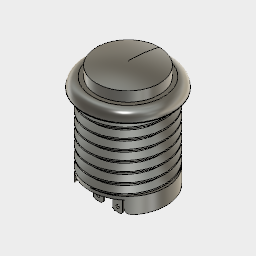
3429 Mini Arcade Button (Autodesk Fusion 360 design; units mm, degrees)
Autodesk Fusion 360 part; units mm, degrees
sketch "main circles" plane through (0, 0, 0) normal (0, 0, 1) x (1, 0, 0)
  circle A0 centre (0, 0) radius 12
  circle A1 centre (0, 0) radius 9.8
  circle A2 centre (0, 0) radius 13.8
  dimension "d1" = 24
  dimension "d2" = 19.6
  dimension "d3" = 27.6
  measures "d1" diameter of A0
  measures "d2" diameter of A1
  measures "d3" diameter of A2
extrude "Extrude1" add sketch "main circles" along normal blind 4.2 contours A1 makes body 1
sketch "curve revolve spline" plane through (0, 0, 0) normal (0, 1, 0) x (1, 0, 0)
  spline S0 degree 5 poles (0, -4.2) (-0.5903, -4.2) (-1.7268, -4.1833) (-3.2991, -4.1084) (-5.1578, -3.9245) (-7.1512, -3.617) (-8.4865, -3.3557) (-9.317, -3.171) (-9.7864, -3.0557) (-10, -3) knots 0 0 0 0 0 0 0.2 0.4 0.6 0.8 1 1 1 1 1 1
  line L0 (-9.8, -4.2) -> (9.8, -4.2)
  line L1 (-9.4578, -3.1414) -> (-10.5422, -2.8586)
  line L2 (1.5, -4.2) -> (-1.5, -4.2)
  line L3 (0, -4.2) -> (0, -6)
  line L4 (0, -6) -> (-11, -6)
  line L5 (-11, -6) -> (-11, -3)
  line L6 (-11, -3) -> (-10, -3)
revolve "Revolve1" cut sketch "curve revolve spline" angle 360 about axis through (0, 0, 1.75) along (0, 0, 1) bodies 1
extrude "Extrude2" add sketch "main circles" against normal blind 3 separate body contours A0 | A1 | A2 makes body 2
fillet "Fillet1" radius 2.8 1 edges at (-12.8661, -4.9903, 0) on bodies 2
extrude "Extrude3" add sketch "main circles" against normal blind 26 from surface at -3 contours A0 bodies 2
thread "Thread1" "ISO Metric profile 24.0 M24x3 6g" major diameter 23.7645 minor diameter 20.3295 pitch 3 angle 60 modelled right hand crest width 0.375 on face at (11.9404, -1.1948, -11.6667) from (0, 0, -3) to (0, 0, -24) crest through (11.8823, 0, -2.8125) on bodies 2
sketch "bottom cutting" plane through (0, 0, 0) normal (1, 0, 0) x (0, 1, 0)
  line L0 (7.75, -35) -> (-7.75, -35)
  line L1 (-7.75, -35) -> (-7.75, -25)
  line L2 (-7.75, -25) -> (7.75, -25)
  line L3 (7.75, -25) -> (7.75, -35)
  line L4 (7.75, -35) -> (-7.75, -25) construction
  line L5 (-7.75, -35) -> (7.75, -25) construction
  line L6 (0, 0) -> (0, -45) construction
  point P0 (0, -30)
  dimension "d15" = 15.5
  dimension "d16" = 10
  dimension "d17" = 30
  measures "d15" distance of L1.end L2.end
  measures "d16" distance of L0.end L1.end
  measures "d17" distance of L6.start P0
extrude "Extrude4" cut sketch "bottom cutting" along normal mid plane 32 bodies 2
fillet "Fillet2" radius 1.5 4 edges at (-7.5025, -7.75, -29) (7.5025, -7.75, -29) (7.5025, 7.75, -29) (-7.5025, 7.75, -29) on bodies 2
ref_plane "WorkPlane1" through (0, 0, -25) normal (0, 0, 1) x (1, 0, 0)
sketch "button housing" plane through (0, 0, -25) normal (0, 0, 1) x (1, 0, 0)
  line L0 (7.25, 6.25) -> (-7.25, 6.25)
  line L1 (-7.25, 6.25) -> (-7.25, -6.25)
  line L2 (-7.25, -6.25) -> (7.25, -6.25)
  line L3 (7.25, -6.25) -> (7.25, 6.25)
  line L4 (7.25, 6.25) -> (-7.25, -6.25) construction
  line L5 (-7.25, 6.25) -> (7.25, -6.25) construction
  dimension "d22" = 12.5
  dimension "d23" = 14.5
  measures "d22" distance of L0.end L1.end
  measures "d23" distance of L1.end L2.end
extrude "Extrude5" add sketch "button housing" along normal blind 6 separate body makes body 3
sketch "electtodes" plane through (0, 0, -25) normal (0, 0, -1) x (1, 0, 0)
  line L0 (7.25, -6.25) -> (7.25, 6.25)
  line L1 (7.25, 6.25) -> (-7.25, 6.25)
  line L2 (-7.25, 6.25) -> (-7.25, -6.25)
  line L3 (-7.25, -6.25) -> (7.25, -6.25)
  line L4 (-4.5, 6.25) -> (-1.5, 6.25)
  line L5 (-1.5, 6.25) -> (-1.5, 5.75)
  line L6 (-1.5, 5.75) -> (-4.5, 5.75)
  line L7 (-4.5, 5.75) -> (-4.5, 6.25)
  line L8 (0, 0) -> (0, 8) construction
  line L9 (0, 0) -> (-15, 0) construction
  line L10 (-4.5, -6.25) -> (-1.5, -6.25)
  line L11 (-1.5, -6.25) -> (-1.5, -5.75)
  line L12 (-1.5, -5.75) -> (-4.5, -5.75)
  line L13 (-4.5, -5.75) -> (-4.5, -6.25)
  line L14 (4.5, 6.25) -> (1.5, 6.25)
  line L15 (1.5, 6.25) -> (1.5, 5.75)
  line L16 (4.5, 5.75) -> (4.5, 6.25)
  line L17 (1.5, 5.75) -> (4.5, 5.75)
  line L18 (4.5, -6.25) -> (1.5, -6.25)
  line L19 (1.5, -6.25) -> (1.5, -5.75)
  line L20 (4.5, -5.75) -> (4.5, -6.25)
  line L21 (1.5, -5.75) -> (4.5, -5.75)
  dimension "d26" = 3
  dimension "d27" = 0.5
  dimension "d28" = 1.5
  measures "d26" distance of L4.start L4.end
  measures "d27" distance of L4.start L6.end
  measures "d28" distance of L5 L8
extrude "Extrude6" add sketch "electtodes" along normal blind 7 contours L3 L18 L19 L20 L21 | L1 L14 L15 L16 L17 | L3 L10 L11 L12 L13 | L1 L4 L5 L6 L7 bodies 3
chamfer "Chamfer1" distance 0.5 angle 45 8 edges at (-4.5, 6, -32) (-1.5, 6, -32) (1.5, 6, -32) (4.5, 6, -32) (-4.5, -6, -32) (-1.5, -6, -32) (1.5, -6, -32) (4.5, -6, -32) on bodies 3
move_body "Move1" bodies 1 2 to x (0, -1, 0) y (1, 0, 0) z (0, 0, 1) at (0, 0, 0)
sketch "Sketch6" plane through (0, -6.25, 0) normal (0, -1, 0) x (1, 0, 0)
  line L0 (4, -32) -> (4.5, -31.5)
  line L1 (4.5, -31.5) -> (4.5, -25)
  line L2 (4.5, -25) -> (7.25, -25)
  line L3 (7.25, -25) -> (7.25, -19)
  line L4 (7.25, -19) -> (-7.25, -19)
  line L5 (-7.25, -19) -> (-7.25, -25)
  line L6 (-7.25, -25) -> (-4.5, -25)
  line L7 (-4.5, -25) -> (-4.5, -31.5)
  line L8 (-4.5, -31.5) -> (-4, -32)
  line L9 (-4, -32) -> (-2, -32)
  line L10 (-2, -32) -> (-1.5, -31.5)
  line L11 (-1.5, -31.5) -> (-1.5, -25)
  line L12 (-1.5, -25) -> (1.5, -25)
  line L13 (1.5, -25) -> (1.5, -31.5)
  line L14 (1.5, -31.5) -> (2, -32)
  line L15 (2, -32) -> (4, -32)
  circle A0 centre (-3, -30.5) radius 0.5
  circle A1 centre (3, -30.5) radius 0.5
  dimension "d32" = 1
  dimension "d33" = 1.5
  dimension "d34" = 1
  dimension "d35" = 1.5
  measures "d32" diameter of A0
  measures "d33" distance of L9 A0.centre
  measures "d34" diameter of A1
  measures "d35" distance of L15 A1.centre
extrude "Extrude7" cut sketch "Sketch6" against normal up to surface (12.5 mm away) contours A0 | A1 bodies 3
named bodies: "cap", "body", "switch"
